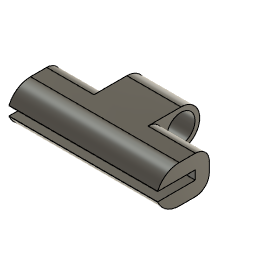
hinge and hinge pin v3 (Autodesk Fusion 360 archive; units mm, degrees)
design "fin hinge v3"
Autodesk Fusion 360 part; units mm, degrees
sketch "Sketch1" plane through (0, 0, 0) normal (1, 0, 0) x (0, 1, 0)
  circle A0 centre (0, 0) radius 2
  circle A1 centre (0, 0) radius 4
  dimension "d1" = 4
  dimension "d2" = 8
  constraint coincident A0.centre A1.centre
  constraint concentric A0 A1
  measures "d1" diameter of A0
  measures "d2" diameter of A1
extrude "Extrude1" add sketch "Sketch1" along normal blind 11.5 makes body 1
sketch "Sketch2" plane through (11.5, 0, 0) normal (1, 0, 0) x (0, 1, 0)
  circle A0 centre (0, 0) radius 2
  circle A1 centre (0, 0) radius 4
  line L0 (0, -4) -> (-15, -4)
  line L1 (-15, -4) -> (-15, -1)
  line L2 (-15, -1) -> (-7, -1)
  line L3 (0, 4) -> (-15, 4)
  line L4 (-15, 4) -> (-15, 1)
  line L5 (-15, 1) -> (-7, 1)
  line L6 (-7, -1) -> (-7, 1)
  constraint coincident A1 L0.start
  constraint tangent A1 L0
  constraint horizontal L0
  constraint perpendicular L0 L1
  constraint perpendicular L1 L2
  constraint coincident A1 L3.start
  constraint tangent A1 L3
  constraint parallel L2 L3
  constraint perpendicular L3 L4
  constraint perpendicular L4 L5
  constraint perpendicular L5 L6
extrude "Extrude2" add sketch "Sketch2" along normal blind 15.859 separate body contours A1 L0 L1 L2 L3 L4 L5 L6 makes body 2
extrude "Extrude3" add 1 faces at (27.359, -12.3333, -2) along direction (-1, 0, 0) blind 43.718 on bodies 2 bodies 2 1
sketch "Sketch3" plane through (27.359, 0, 0) normal (1, 0, 0) x (0, 1, 0)
  line L0 (0, 4) -> (-15, 4)
  line L1 (-15, 4) -> (-15, 1)
  line L2 (-15, 1) -> (-7, 1)
  line L3 (-7, 1) -> (-7, -1)
  line L4 (-7, -1) -> (-15, -1)
  line L5 (-15, -1) -> (-15, -4)
  line L6 (-15, -4) -> (0, -4)
  arc A0 (0, 4) -> (0, -4) centre (0, 0) ccw
  line L7 (-4, 0) -> (-4, -4)
  line L8 (-4, 0) -> (-4, 4)
  constraint midpoint A0 L7.start
  constraint coincident L6 L7.end
  constraint tangent A0 L7
  constraint perpendicular L6 L7
  constraint coincident L0 L8.end
  constraint tangent A0 L8
  constraint perpendicular L0 L8
extrude "Extrude4" cut sketch "Sketch3" against normal blind 15.859 contours L0 A0 L8 | L6 A0 L7 bodies 2
sketch "Sketch4" plane through (-16.359, 0, 0) normal (-1, 0, 0) x (0, -1, 0)
  line L0 (15, 4) -> (0, 4)
  arc A0 (0, -4) -> (0, 4) centre (0, 0) ccw
  line L1 (0, -4) -> (15, -4)
  line L2 (15, -4) -> (15, -1)
  line L3 (15, -1) -> (7, -1)
  line L4 (7, -1) -> (7, 1)
  line L5 (7, 1) -> (15, 1)
  line L6 (15, 1) -> (15, 4)
  line L7 (4, 0) -> (4, 4)
  line L8 (4, 0) -> (4, -4)
  constraint midpoint A0 L7.start
  constraint coincident L0 L7.end
  constraint tangent A0 L7
  constraint perpendicular L0 L7
  constraint coincident L1 L8.end
  constraint tangent A0 L8
  constraint perpendicular L1 L8
extrude "Extrude5" cut sketch "Sketch4" against normal blind 16.359 contours L0 A0 L7 | A0 L1 L8 bodies 2
fillet "Fillet1" radius 3 4 edges at (19.4295, -4, 4) (-8.1795, -4, 4) (-8.1795, -4, -4) (19.4295, -4, -4) on bodies 2
fillet "Fillet2" radius 5 2 edges at (5.5, -15, 4) (5.5, -15, -4) on bodies 2
extrude "Extrude6" cut 1 faces at (-16.359, -8.1391, -3) along direction (1, 0, 0) blind 6.303 on bodies 2 bodies 2
extrude "Extrude7" cut 1 faces at (27.359, -8.1391, -3) along direction (-1, 0, 0) blind 5.533 on bodies 2 bodies 2
extrude "Extrude8" cut 1 faces at (21.826, -8.1391, -3) along direction (-1, 0, 0) blind 0.27 on bodies 2 bodies 2
extrude "Extrude9" add 1 faces at (11.0187, -12.3333, -1) along direction (0, 0, 1) blind 0.05 on bodies 2 bodies 2
extrude "Extrude10" add 1 faces at (11.0187, -12.3333, 1) along direction (0, 0, -1) blind 0.05 on bodies 2 bodies 2
move_face "OffsetFaces1" offset -1 1 faces at (7.6667, 1.9975, -0.0997) on bodies 2
